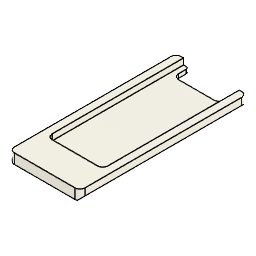
mriya-niceview-holder-fdm-v1.01 (Autodesk Fusion 360 design; units mm, degrees)
Autodesk Fusion 360 part; units mm, degrees
sketch "mriya-niceview-holder" plane through (0, 0, 0) normal (0, 0, 1) x (1, 0, 0)
  line L0 (-20.8, 9.9) -> (-9.8, 9.9)
  line L1 (-9.8, 9.9) -> (-9.8, 36.9)
  line L2 (-22.3, 3.9) -> (-22.3, 36.9)
  line L3 (-20.8, 9.9) -> (-20.8, 36.9)
  line L4 (-8.3, 36.9) -> (-8.3, 3.9)
  line L5 (-22.3, 36.9) -> (-19.8, 36.9)
  line L6 (-22.3, 3.9) -> (-8.3, 3.9)
  arc A0 (-19.8, 34.9) -> (-18.8, 33.9) centre (-18.8, 34.9) ccw
  line L7 (-10.8, 36.9) -> (-8.3, 36.9)
  arc A1 (-11.8, 33.9) -> (-10.8, 34.9) centre (-11.8, 34.9) ccw
  line L8 (-10.8, 34.9) -> (-10.8, 36.9)
  line L9 (-18.8, 33.9) -> (-11.8, 33.9)
  line L10 (-19.8, 34.9) -> (-19.8, 36.9)
  constraint perpendicular L4 L5
  constraint coincident L3.end L5
  constraint coincident L1.end L5
  constraint perpendicular L1 L9
  constraint coincident L7.start L5
  constraint collinear L5 L7
  constraint tangent A0 L10
  constraint tangent A0 L9
  constraint tangent A1 L8
  constraint tangent A1 L9
extrude "Extrude1" add sketch "mriya-niceview-holder" along normal blind 2 contours L0 L1 L2 L3 L4 L5 L6 L7
extrude "Extrude2" add sketch "mriya-niceview-holder" along normal blind 0.8 contours L0 L1 L3 L5 A0 L7 A1 L8 L9 L10
chamfer "Chamfer4" distance 0.6 angle 45 2 edges at (-22.3, 20.4, 0) (-8.3, 20.4, 0)
fillet "Fillet1" radius 1 4 edges at (-8.3, 3.9, 1) (-22.3, 3.9, 1) (-8.3, 36.9, 1) (-22.3, 36.9, 1)
fillet "Fillet2" radius 0.5 2 edges at (-10.8, 36.9, 0.4) (-19.8, 36.9, 0.4)
fillet "Fillet3" radius 1 2 edges at (-20.8, 9.9, 1.4) (-9.8, 9.9, 1.4)
